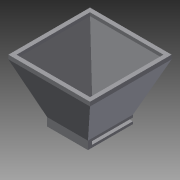
# Autodesk Inventor part: funnel_
Saved by Autodesk Inventor 2014 SP2 (Build 180246200, 246)
## iProperties
Created: 2015-11-28
Part Number: funnel_
Material: Generic
Document SubType Name: Modeling
Designer: schrluka
Density: 1 g/cm^3
Appearance: Default
Author: schrluka
Autodesk Inventor part; units mm, degrees
ref_plane "YZ Plane" through (0, 0, 0) normal (1, 0, 0) x (0, 1, 0)
ref_plane "XZ Plane" through (0, 0, 0) normal (0, 1, 0) x (-1, 0, 0)
sketch "Sketch1" plane through (0, 0, 0) normal (0, 0, 1) x (1, 0, 0)
  line L0 (-25, -27.5) -> (25, -27.5)
  line L1 (25, -27.5) -> (25, 27.5)
  line L2 (25, 27.5) -> (-25, 27.5)
  line L3 (-25, 27.5) -> (-25, -27.5)
  line L4 (-25, -27.5) -> (25, 27.5) construction
  line L5 (25, -27.5) -> (-25, 27.5) construction
  point P0 (0, 0)
  dimension "d0" = 50
  dimension "d1" = 55
  constraints: 12 end point, 2 midpoint, 2 parallel, 1 horizontal, 1 perpendicular
  measures "d0" distance of L2.end L1.end
  measures "d1" distance of L1.end L0.end
extrude "Extrusion1" add sketch "Sketch1" along normal blind 10
ref_plane "Work Plane1" through (0, 0, 70) normal (0, 0, 1) x (1, 0, 0)
sketch "Sketch3" plane through (0, 0, 70) normal (0, 0, 1) x (1, 0, 0)
  line L0 (-50, -50) -> (50, -50)
  line L1 (50, -50) -> (50, 50)
  line L2 (50, 50) -> (-50, 50)
  line L3 (-50, 50) -> (-50, -50)
  line L4 (-50, -50) -> (50, 50) construction
  line L5 (50, -50) -> (-50, 50) construction
  line L6 (-42.5, -42.5) -> (42.5, 42.5) construction
  line L7 (42.5, -42.5) -> (-42.5, 42.5) construction
  point P0 (0, 0)
  dimension "d9" = 100
  dimension "d10" = 100
  constraints: 16 end point, 4 midpoint, 2 parallel, 1 horizontal, 1 perpendicular
  measures "d9" distance of L2.end L1.end
  measures "d10" distance of L1.end L0.end
extrude "Extrusion3" add sketch "Sketch3" along normal blind 5
loft "Loft1" add section 1 edges at (0, -27.5, 10) (25, 0, 10) (0, 27.5, 10) (-25, 0, 10) section 2 edges at (0, -50, 70) (-50, 0, 70) (0, 50, 70) (50, 0, 70)
shell "Shell2" thickness 5 removed faces 1 at (-16.6667, 16.6667, 75)
sketch "Sketch4" plane through (25, -27.5, 0) normal (1, 0, 0) x (0, 0, -1)
  line L0 (0, 55) -> (-10, 55) projected
  line L1 (0, 0) -> (-10, 0) projected
  line L2 (-3, 55) -> (-7, 55)
  line L3 (-7, 55) -> (-7, 5)
  line L4 (-7, 5) -> (-3, 5)
  line L5 (-3, 5) -> (-3, 55)
  point P0 (0, 27.5)
  dimension "d28" = 4
  dimension "d29" = 3
  dimension "d30" = 5
  constraints: 8 end point, 2 parallel, 1 horizontal, 1 perpendicular, 1 point on line
  measures "d28" distance of L2.start L2.end
  measures "d29" distance of L2.end L0.end
  measures "d30" distance between parallel lines of L4 L1
extrude "Extrusion4" cut sketch "Sketch4" against normal up to surface (45 mm away)
sketch "Sketch5" plane through (0, 0, 0) normal (0, 0, -1) x (-1, 0, 0)
  line L0 (-20, 22.5) -> (20, 22.5) construction
  line L1 (20, 22.5) -> (-20, 22.5) projected
  line L2 (20, -22.5) -> (20, 52.5) construction
  arc A0 (-20, -10.9429) -> (20, -22.5) centre (20, 52.5) ccw
  line L3 (20, -22.5) -> (20, 22.5)
  line L4 (-20, 22.5) -> (-20, -22.5) projected
  line L5 (-20, 22.5) -> (-20, -22.5) projected
  line L6 (-20, -22.5) -> (-20, -22.535) projected
  line L7 (-20, -22.535) -> (-20, 22.535) projected
  line L8 (-20, 22.5) -> (-20, 22.535) projected
  line L9 (-20, -10.9429) -> (-20, 22.5)
  line L10 (20, 22.5) -> (-20, 22.5)
  point P0 (0, 0)
  dimension "d31" = 75
  constraints: 8 end point, 2 collinear, 2 perpendicular, 2 point on circle, 1 centre point, 1 coincident, 1 point on line
  measures "d31" distance of L2.start L2.end
extrude "Extrusion5" cut sketch "Sketch5" against normal through all
body "Solid1"
